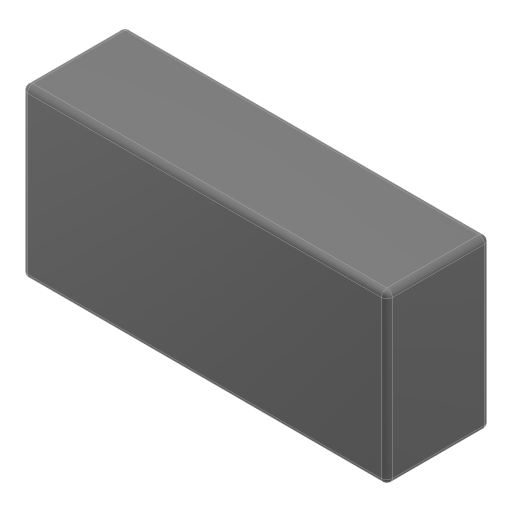
# Autodesk Inventor part: Zeee6S22Ah
Saved by Autodesk Inventor 2024 (Build 280153000, 153)
## iProperties
Created: 2025-11-20
Part Number: Zeee6S22Ah
Material: Plastic, Opaque Black
Document SubType Name: Modeling
Designer: gaoet
Density: 0.952 g/cm^3
Appearance: Smooth - Black
Author: gaoet
Autodesk Inventor part; units mm, degrees
ref_plane "YZ Plane" through (0, 0, 0) normal (1, 0, 0) x (0, 1, 0)
ref_plane "XZ Plane" through (0, 0, 0) normal (0, 1, 0) x (-1, 0, 0)
ref_plane "XY Plane" through (0, 0, 0) normal (0, 0, 1) x (1, 0, 0)
sketch "Sketch1" plane through (0, 0, 0) normal (0, 0, 1) x (1, 0, 0)
  line L0 (-99, -45.5) -> (99, -45.5)
  line L1 (99, -45.5) -> (99, 45.5)
  line L2 (99, 45.5) -> (-99, 45.5)
  line L3 (-99, 45.5) -> (-99, -45.5)
  line L4 (-99, -45.5) -> (99, 45.5) construction
  line L5 (99, -45.5) -> (-99, 45.5) construction
  point P0 (0, 0)
  dimension "d0" = 198
  dimension "d1" = 91
  constraints: 12 end point, 2 midpoint, 2 parallel, 1 horizontal, 1 perpendicular
  measures "d0" distance of L2.end L1.end
  measures "d1" distance of L1.end L0.end
extrude "Extrusion1" add sketch "Sketch1" along normal blind 56
fillet "Fillet1" radius 3 12 edges at (0, 45.5, 56) (99, 0, 56) (99, 0, 0) (99, 45.5, 28) (0, 45.5, 0) (-99, 45.5, 28) (-99, 0, 56) (-99, 0, 0) (-99, -45.5, 28) (0, -45.5, 56) (99, -45.5, 28) (0, -45.5, 0)
body "Solid1"
